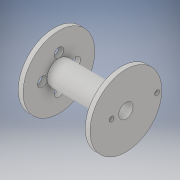
# Autodesk Inventor part: Spool1
Saved by Autodesk Inventor 2019 (Build 230136000, 136)
## iProperties
Created: 2019-01-14
Part Number: Spool1
Material: Generic
Document SubType Name: Modeling
Designer: Kepler
Density: 1 g/cm^3
Appearance: Default
Author: Kepler
Autodesk Inventor part; units mm, degrees
ref_plane "YZ Plane" through (0, 0, 0) normal (1, 0, 0) x (0, 1, 0)
ref_plane "XZ Plane" through (0, 0, 0) normal (0, 1, 0) x (-1, 0, 0)
ref_plane "XY Plane" through (0, 0, 0) normal (0, 0, 1) x (1, 0, 0)
sketch "Sketch1" plane through (0, 0, 0) normal (0, 0, 1) x (1, 0, 0)
  line L0 (0, 0) -> (2, 0)
  line L1 (2, 0) -> (2, 10)
  line L2 (2, 10) -> (28, 10)
  line L3 (28, 10) -> (28, 0)
  line L4 (28, 0) -> (30, 0)
  line L5 (30, 0) -> (30, 12)
  line L6 (30, 12) -> (0, 12)
  line L7 (0, 12) -> (0, 0)
  line L8 (30, 15) -> (0, 15)
  dimension "d0" = 2
  dimension "d1" = 10
  dimension "d2" = 26
  dimension "d3" = 2
  dimension "d4" = 12
  dimension "d5" = 3
  dimension "d6" = 30
  constraints: 18 end point, 6 perpendicular, 4 point on line, 1 horizontal, 1 parallel
  measures "d0" distance of L0.start L0.end
  measures "d1" distance of L0.end L1.end
  measures "d2" distance of L1.end L2.end
  measures "d3" distance of L3.end L4.end
  measures "d4" distance of L4.end L5.end
  measures "d5" distance of L5.end L8.start
  measures "d6" distance between parallel lines of L5 L7
revolve "Revolution1" add sketch "Sketch1" angle 360 about axis through (30, 15, 0) along (-1, 0, 0)
sketch "Sketch2" plane through (0, 15, 0) normal (-1, 0, 0) x (0, 0, 1)
  circle A0 centre (7, 0) radius 2
  circle A1 centre (-7, 0) radius 2
  circle A2 centre (0, 7) radius 2
  circle A3 centre (0, -7) radius 2
  point P0 (0, -15)
  point P1 (0, 0)
  dimension "d8" = 4
  dimension "d10" = 4
  dimension "d13" = 4
  dimension "d14" = 4
  dimension "d17" = 7
  dimension "d18" = 7
  dimension "d19" = 7
  dimension "d20" = 7
  constraints: 4 centre point
  measures "d8" diameter of A0
  measures "d10" diameter of A1
  measures "d13" diameter of A2
  measures "d14" diameter of A3
  measures "d17" distance of point (0, 0) A1.centre
  measures "d18" distance of point (0, 0) A2.centre
  measures "d19" distance of point (0, 0) A0.centre
  measures "d20" distance of point (0, 0) A3.centre
sketch "Sketch3" plane through (0, 15, 0) normal (-1, 0, 0) x (0, 0, 1)
  point P0 (0, -15)
extrude "Extrusion1" cut sketch "Sketch2" against normal blind 2
sketch "Sketch4" plane through (30, 15, 0) normal (1, 0, 0) x (0, 0, -1)
  circle A0 centre (13, 0) radius 1
  circle A1 centre (-6, 0) radius 1
  point P0 (0, -15)
  point P1 (0, 0)
  dimension "d23" = 2
  dimension "d24" = 2
  dimension "d25" = 6
  dimension "d26" = 13
  constraints: 2 centre point, 1 other
  measures "d23" diameter of A0
  measures "d24" diameter of A1
  measures "d25" distance of point (0, 0) A1.centre
  measures "d26" distance of point (0, 0) A0.centre
extrude "Extrusion2" cut sketch "Sketch4" against normal blind 2
body "Solid1"
